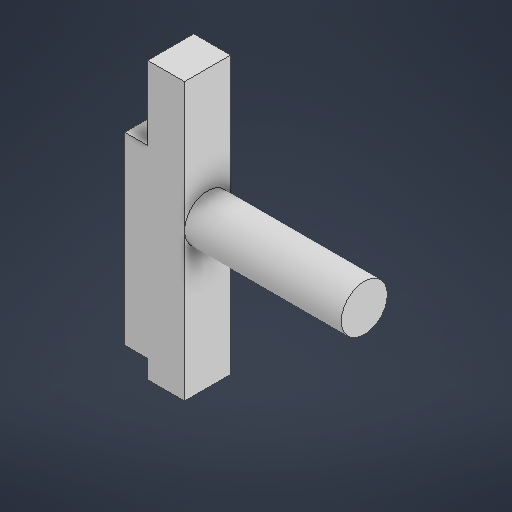
# Autodesk Inventor part: contact_axis
Saved by Autodesk Inventor 2027 (Build 310192000, 192)
## iProperties
Created: 2026-05-24
Part Number: contact_axis
Material: Generic
Document SubType Name: Modeling
Designer: alexy
Density: 1 g/cm^3
Appearance: Default
Author: alexy
Autodesk Inventor part; units mm, degrees
ref_plane "YZ Plane" through (0, 0, 0) normal (1, 0, 0) x (0, 1, 0)
ref_plane "XZ Plane" through (0, 0, 0) normal (0, 1, 0) x (-1, 0, 0)
ref_plane "XY Plane" through (0, 0, 0) normal (0, 0, 1) x (1, 0, 0)
sketch "Sketch1" plane through (0, 0, 0) normal (0, 0, 1) x (1, 0, 0)
  line L0 (0, 0) -> (4, 0)
  line L1 (4, 0) -> (4, 30)
  line L2 (4, 30) -> (0, 30)
  line L3 (0, 30) -> (0, 0)
  line L4 (-2.5, 22) -> (0, 22)
  line L5 (0, 22) -> (0, 2)
  line L6 (0, 2) -> (-2.5, 2)
  line L7 (-2.5, 2) -> (-2.5, 22)
  point P0 (-1.25, 2)
  point P1 (0, 22)
  dimension "d0" = 2.5
  dimension "d1" = 20
  dimension "d2" = 30
  dimension "d3" = 4
  dimension "d4" = 2
  constraints: 16 end point, 4 parallel, 2 horizontal, 2 perpendicular, 1 midpoint, 1 point on line
  measures "d0" distance of L5.end L6.end
  measures "d1" distance of L6.end L4.start
  measures "d2" distance of L0.end L1.end
  measures "d3" distance of L0.start L0.end
  measures "d4" vertical distance of L0.start point (-1.25, 2)
extrude "Extrusion1" add sketch "Sketch1" along normal blind 5
sketch "Sketch2" plane through (4, 0, 0) normal (1, 0, 0) x (0, 0, -1)
  circle A0 centre (-2.5, 16) radius 2.5
  line L0 (0, 0) -> (0, 30) projected
  line L1 (0, 30) -> (-5, 30) projected
  point P0 (-2.5, 30)
  dimension "d7" = 14
  constraints: 1 centre point, 1 midpoint, 1 tangent, 1 vertical alignment
  measures "d7" distance from line of L1 A0.centre
extrude "Extrusion2" add sketch "Sketch2" along normal blind 17
body "Solid1"
